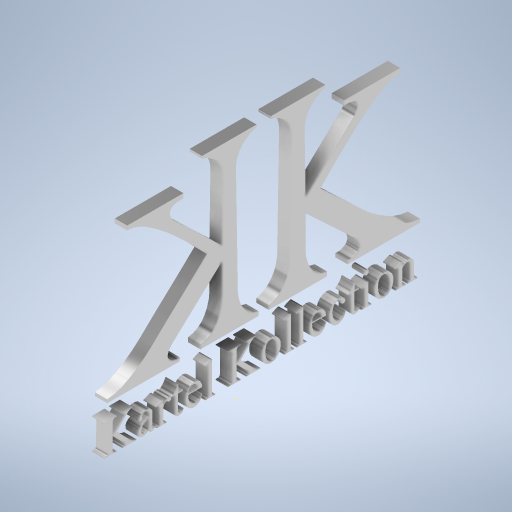
# Autodesk Inventor part: Kartel
Saved by Autodesk Inventor 2024 (Build 280153000, 153)
## iProperties
Created: 2024-08-29
Part Number: Kartel
Material: Genérico
Document SubType Name: Modeling
Designer: aless
Density: 1 g/cm^3
Appearance: Valor por defecto
Author: aless
Autodesk Inventor part; units mm, degrees
ref_plane "YZ Plane" through (0, 0, 0) normal (1, 0, 0) x (0, 1, 0)
ref_plane "XZ Plane" through (0, 0, 0) normal (0, 1, 0) x (-1, 0, 0)
ref_plane "XY Plane" through (0, 0, 0) normal (0, 0, 1) x (1, 0, 0)
sketch "Boceto1" plane through (0, 0, 0) normal (1, 0, 0) x (0, 1, 0)
  line L0 (223.396, 155.4576) -> (223.396, -178.2855) construction
  line L1 (223.396, -178.2855) -> (-110.3471, -178.2855) construction
  line L2 (-110.3471, -178.2855) -> (-110.3471, 155.4576) construction
  line L3 (-110.3471, 155.4576) -> (223.396, 155.4576) construction
  line L4 (59.7919, 115.7755) -> (59.7919, 56.339)
  line L5 (59.7919, 56.339) -> (62.7617, 56.339)
  arc A0 (64.6613, 64.2665) -> (62.7617, 56.339) centre (72.9401, 58.0914) ccw
  arc A1 (69.206, 66.1601) -> (64.6613, 64.2665) centre (68.5307, 61.3804) ccw
  arc A2 (72.0463, 65.151) -> (69.206, 66.1601) centre (68.1498, 58.6851) ccw
  arc A3 (76.4937, 61.3804) -> (72.0463, 65.151) centre (62.6533, 49.5641) ccw
  line L6 (76.4937, 61.3804) -> (113.4232, 21.7725)
  line L7 (113.4232, 21.7725) -> (88.008, 21.7725)
  arc A4 (71.6292, 26.2448) -> (88.008, 21.7725) centre (88.008, 54.0005) ccw
  arc A5 (63.3483, 39.331) -> (71.6292, 26.2448) centre (80.259, 40.8688) ccw
  line L8 (63.3483, 39.331) -> (59.7919, 39.331)
  line L9 (59.7919, 39.331) -> (59.7919, -8.3342)
  line L10 (59.7919, -8.3342) -> (63.1296, -8.3342)
  arc A6 (68.7765, 1.9584) -> (63.1296, -8.3342) centre (81.2261, -11.5671) ccw
  arc A7 (78.8624, 7.5023) -> (68.7765, 1.9584) centre (85.0773, -15.7512) ccw
  arc A8 (85.9805, 8.7127) -> (78.8624, 7.5023) centre (88.9297, -30.165) ccw
  line L11 (85.9805, 8.7127) -> (173.9872, 10.2175)
  arc A9 (184.4936, 7.5023) -> (173.9872, 10.2175) centre (174.3349, -10.1219) ccw
  arc A10 (194.6699, -6.6902) -> (184.4936, 7.5023) centre (173.2187, -11.3266) ccw
  line L12 (194.6699, -6.6902) -> (196.5458, -6.6902)
  line L13 (196.5458, -6.6902) -> (196.5458, 38.0381)
  line L14 (196.5458, 38.0381) -> (194.6699, 38.0381)
  arc A11 (186.9942, 25.7984) -> (194.6699, 38.0381) centre (168.397, 45.9875) ccw
  arc A12 (178.5832, 21.5693) -> (186.9942, 25.7984) centre (172.938, 43.2753) ccw
  arc A13 (175.6544, 21.0123) -> (178.5832, 21.5693) centre (172.938, 43.2753) ccw
  line L15 (175.6544, 21.0123) -> (124.7977, 21.7725)
  line L16 (124.7977, 21.7725) -> (161.7029, 60.4981)
  arc A14 (168.397, 64.5278) -> (161.7029, 60.4981) centre (170.5786, 53.329) ccw
  arc A15 (173.3252, 61.0636) -> (168.397, 64.5278) centre (168.6661, 59.673) ccw
  arc A16 (173.9954, 53.3315) -> (173.3252, 61.0636) centre (154.9336, 55.5745) ccw
  line L17 (173.9954, 53.3315) -> (177.7934, 53.3315)
  line L18 (177.7934, 53.3315) -> (177.7934, 99.4261)
  line L19 (177.7934, 99.4261) -> (174.3349, 99.4261)
  arc A17 (172.6788, 91.0496) -> (174.3349, 99.4261) centre (150.1011, 99.8653) ccw
  arc A18 (166.5655, 79.9474) -> (172.6788, 91.0496) centre (127.5163, 108.6838) ccw
  arc A19 (152.2652, 61.8267) -> (166.5655, 79.9474) centre (37.6495, 166.9808) ccw
  arc A20 (124.9813, 34.0587) -> (152.2652, 61.8267) centre (-154.1606, 335.6217) ccw
  arc A21 (95.3768, 65.5592) -> (124.9813, 34.0587) centre (1804.822, 1642.4536) ccw
  line L20 (95.3768, 65.5592) -> (82.3934, 79.0506)
  arc A22 (68.1498, 98.3694) -> (82.3934, 79.0506) centre (151.211, 144.6993) ccw
  arc A23 (62.5253, 115.7755) -> (68.1498, 98.3694) centre (101.6273, 118.7989) ccw
  line L21 (59.7919, 115.7755) -> (62.5253, 115.7755)
  line L22 (59.7919, -140.8555) -> (59.7919, -81.419)
  line L23 (59.7919, -81.419) -> (62.7617, -81.419)
  arc A24 (62.7617, -81.419) -> (64.6613, -89.3466) centre (72.9401, -83.1714) ccw
  arc A25 (64.6613, -89.3466) -> (69.206, -91.2401) centre (68.5307, -86.4604) ccw
  arc A26 (69.206, -91.2401) -> (72.0463, -90.231) centre (68.1498, -83.7652) ccw
  arc A27 (72.0463, -90.231) -> (76.4937, -86.4604) centre (62.6533, -74.6442) ccw
  line L24 (76.4937, -86.4604) -> (113.4232, -46.8526)
  line L25 (113.4232, -46.8526) -> (88.008, -46.8526)
  arc A28 (88.008, -46.8526) -> (71.6292, -51.3249) centre (88.008, -79.0805) ccw
  arc A29 (71.6292, -51.3249) -> (63.3483, -64.411) centre (80.259, -65.9489) ccw
  line L26 (63.3483, -64.411) -> (59.7919, -64.411)
  line L27 (59.7919, -64.411) -> (59.7919, -16.7458)
  line L28 (59.7919, -16.7458) -> (63.1296, -16.7458)
  arc A30 (63.1296, -16.7458) -> (68.7765, -27.0385) centre (81.2261, -13.513) ccw
  arc A31 (68.7765, -27.0385) -> (78.8624, -32.5823) centre (85.0773, -9.3289) ccw
  arc A32 (78.8624, -32.5823) -> (85.9805, -33.7928) centre (88.9297, 5.0849) ccw
  line L29 (85.9805, -33.7928) -> (173.9872, -35.2975)
  arc A33 (173.9872, -35.2975) -> (184.4936, -32.5823) centre (174.3349, -14.9582) ccw
  arc A34 (184.4936, -32.5823) -> (194.6699, -18.3898) centre (173.2187, -13.7535) ccw
  line L30 (194.6699, -18.3898) -> (196.5458, -18.3898)
  line L31 (196.5458, -18.3898) -> (196.5458, -63.1181)
  line L32 (196.5458, -63.1181) -> (194.6699, -63.1181)
  arc A35 (194.6699, -63.1181) -> (186.9942, -50.8784) centre (168.397, -71.0676) ccw
  arc A36 (186.9942, -50.8784) -> (178.5832, -46.6493) centre (172.938, -68.3554) ccw
  arc A37 (178.5832, -46.6493) -> (175.6544, -46.0923) centre (172.938, -68.3554) ccw
  line L33 (175.6544, -46.0923) -> (124.7977, -46.8526)
  line L34 (124.7977, -46.8526) -> (161.7029, -85.5781)
  arc A38 (161.7029, -85.5781) -> (168.397, -89.6078) centre (170.5786, -78.409) ccw
  arc A39 (168.397, -89.6078) -> (173.3252, -86.1436) centre (168.6661, -84.7531) ccw
  arc A40 (173.3252, -86.1436) -> (173.9954, -78.4115) centre (154.9336, -80.6545) ccw
  line L35 (173.9954, -78.4115) -> (177.7934, -78.4115)
  line L36 (177.7934, -78.4115) -> (177.7934, -124.5062)
  line L37 (177.7934, -124.5062) -> (174.3349, -124.5062)
  arc A41 (174.3349, -124.5062) -> (172.6788, -116.1296) centre (150.1011, -124.9454) ccw
  arc A42 (172.6788, -116.1296) -> (166.5655, -105.0274) centre (127.5163, -133.7638) ccw
  arc A43 (166.5655, -105.0274) -> (152.2652, -86.9067) centre (37.6495, -192.0609) ccw
  arc A44 (152.2652, -86.9067) -> (124.9813, -59.1387) centre (-154.1606, -360.7017) ccw
  arc A45 (124.9813, -59.1387) -> (95.3768, -90.6393) centre (1804.822, -1667.5336) ccw
  line L38 (95.3768, -90.6393) -> (82.3934, -104.1306)
  arc A46 (82.3934, -104.1306) -> (68.1498, -123.4494) centre (151.211, -169.7794) ccw
  arc A47 (68.1498, -123.4494) -> (62.5253, -140.8555) centre (101.6273, -143.879) ccw
  line L39 (59.7919, -140.8555) -> (62.5253, -140.8555)
  arc A48 (38.0866, 85.5965) -> (35.5198, 87.3022) centre (35.8691, 85.0436) ccw
  arc A49 (36.8943, 82.0362) -> (38.0866, 85.5965) centre (34.9982, 84.651) ccw
  arc A50 (34.9982, 81.6224) -> (36.8943, 82.0362) centre (35.1843, 85.3209) ccw
  line L40 (34.9982, 81.6224) -> (32.9082, 81.6224)
  arc A51 (32.9082, 81.6224) -> (29.9007, 88.3728) centre (12.5435, 76.5945) ccw
  arc A52 (29.9007, 88.3728) -> (24.2156, 90.5789) centre (25.542, 85.5688) ccw
  arc A53 (24.2156, 90.5789) -> (21.9144, 84.651) centre (25.5922, 86.6339) ccw
  arc A54 (21.9144, 84.651) -> (24.2156, 81.6224) centre (39.6273, 95.7211) ccw
  arc A55 (23.3542, 81.4464) -> (24.2156, 81.6224) centre (23.3384, 83.7198) ccw
  arc A56 (23.3542, 81.4464) -> (21.6972, 78.3656) centre (23.3681, 79.4529) ccw
  arc A57 (21.6972, 78.3656) -> (24.0265, 75.8904) centre (29.735, 83.5959) ccw
  line L41 (24.0265, 75.8904) -> (24.977, 75.8904)
  arc A58 (23.7493, 77.1285) -> (24.977, 75.8904) centre (26.642, 78.769) ccw
  arc A59 (24.5577, 78.769) -> (23.7493, 77.1285) centre (24.9399, 77.5613) ccw
  line L42 (24.5577, 78.769) -> (34.6579, 78.769)
  arc A60 (34.6579, 78.769) -> (36.5914, 78.9939) centre (35.1641, 82.8408) ccw
  arc A61 (36.5914, 78.9939) -> (38.1207, 80.244) centre (34.9292, 82.5878) ccw
  arc A62 (38.1207, 80.244) -> (39.1394, 82.8837) centre (33.769, 83.4399) ccw
  arc A63 (39.1394, 82.8837) -> (39.1713, 85.2713) centre (22.5869, 84.2987) ccw
  arc A64 (39.1713, 85.2713) -> (37.0863, 89.3907) centre (33.3893, 84.9322) ccw
  arc A65 (37.0863, 89.3907) -> (34.4999, 89.9538) centre (35.1334, 86.6421) ccw
  arc A66 (34.4999, 89.9538) -> (33.5882, 87.7349) centre (34.6764, 88.5846) ccw
  arc A67 (33.5882, 87.7349) -> (35.5198, 87.3022) centre (34.8398, 88.794) ccw
  line L43 (31.9452, 81.6224) -> (25.277, 81.6224)
  arc A68 (23.3681, 85.4937) -> (25.277, 81.6224) centre (28.802, 85.7668) ccw
  arc A69 (25.3794, 87.7349) -> (23.3681, 85.4937) centre (25.602, 85.5121) ccw
  arc A70 (29.6078, 86.2704) -> (25.3794, 87.7349) centre (26.3335, 83.6533) ccw
  arc A71 (31.9452, 81.6224) -> (29.6078, 86.2704) centre (15.4947, 76.2615) ccw
  line L44 (21.6124, 75.123) -> (21.6124, 66.9623)
  line L45 (21.6124, 66.9623) -> (22.1976, 66.9623)
  arc A72 (23.8036, 69.605) -> (22.1976, 66.9623) centre (24.42, 67.421) ccw
  arc A73 (25.0547, 69.7635) -> (23.8036, 69.605) centre (24.8387, 66.4503) ccw
  line L46 (25.0547, 69.7635) -> (33.686, 69.7635)
  arc A74 (36.3591, 68.1202) -> (33.686, 69.7635) centre (33.1882, 65.9579) ccw
  arc A75 (36.4721, 66.3785) -> (36.3591, 68.1202) centre (35.0858, 67.1631) ccw
  arc A76 (36.4721, 66.3785) -> (36.1827, 63.6509) centre (37.3383, 64.9074) ccw
  arc A77 (36.1827, 63.6509) -> (38.546, 63.7009) centre (37.3383, 64.9074) ccw
  arc A78 (38.546, 63.7009) -> (38.8749, 66.6601) centre (36.4741, 65.429) ccw
  arc A79 (38.8749, 66.6601) -> (35.5198, 69.4394) centre (32.3716, 62.2244) ccw
  arc A80 (35.5198, 69.7635) -> (35.5198, 69.4394) centre (35.6479, 69.6014) ccw
  line L47 (35.5198, 69.7635) -> (39.1779, 69.7635)
  line L48 (39.1779, 69.7635) -> (39.1779, 71.1938)
  line L49 (39.1779, 71.1938) -> (37.1902, 75.9142)
  line L50 (37.1902, 75.9142) -> (36.655, 75.9142)
  arc A81 (36.2727, 73.4734) -> (36.655, 75.9142) centre (34.9055, 74.9378) ccw
  arc A82 (35.4631, 73.138) -> (36.2727, 73.4734) centre (35.236, 74.8315) ccw
  line L51 (35.4631, 73.138) -> (23.8203, 72.7044)
  arc A83 (22.4058, 73.9437) -> (23.8203, 72.7044) centre (23.8947, 74.2162) ccw
  line L52 (22.4058, 73.9437) -> (22.3522, 75.123)
  line L53 (22.3522, 75.123) -> (21.6124, 75.123)
  line L54 (38.1207, 62.9191) -> (37.6239, 62.9191)
  arc A84 (38.1207, 62.9191) -> (44.215, 58.0655) centre (46.9664, 67.7732) ccw
  line L55 (44.215, 58.0655) -> (44.215, 57.4949)
  line L56 (44.215, 57.4949) -> (38.546, 57.4949)
  line L57 (38.546, 57.4949) -> (38.546, 53.7418)
  line L58 (38.546, 53.7418) -> (37.6239, 53.7418)
  line L59 (37.6239, 53.7418) -> (37.6239, 57.6656)
  line L60 (37.6239, 57.6656) -> (25.9541, 57.6656)
  arc A85 (25.9541, 57.6656) -> (24.0759, 57.0554) centre (25.6588, 55.3787) ccw
  arc A86 (24.0759, 57.0554) -> (24.0759, 54.3896) centre (25.4621, 55.7225) ccw
  arc A87 (24.0759, 54.3896) -> (24.977, 53.7418) centre (26.9231, 57.3995) ccw
  line L61 (24.977, 53.7418) -> (24.977, 53.123)
  arc A88 (21.9823, 58.8624) -> (24.977, 53.123) centre (25.6258, 57.1125) ccw
  arc A89 (25.4621, 60.3359) -> (21.9823, 58.8624) centre (24.8526, 56.9298) ccw
  line L62 (25.4621, 60.3359) -> (37.6239, 60.3359)
  line L63 (37.6239, 60.3359) -> (37.6239, 62.9191)
  line L64 (32.3716, 49.3309) -> (32.3716, 37.9509)
  arc A90 (32.3716, 37.9509) -> (38.546, 41.305) centre (32.9408, 44.2631) ccw
  arc A91 (38.546, 41.305) -> (38.8321, 46.6) centre (32.9408, 44.2631) ccw
  arc A92 (38.8321, 46.6) -> (33.9054, 51.0491) centre (31.015, 42.8962) ccw
  arc A93 (33.9054, 51.0491) -> (25.4621, 50.8397) centre (29.9574, 39.913) ccw
  arc A94 (25.4621, 50.8397) -> (21.373, 45.7244) centre (28.4076, 44.293) ccw
  arc A95 (21.373, 45.7244) -> (24.6427, 39.0414) centre (27.4289, 44.546) ccw
  arc A96 (24.6427, 39.0414) -> (27.8582, 37.816) centre (29.5234, 47.0167) ccw
  line L65 (27.8582, 37.816) -> (28.1489, 38.3827)
  arc A97 (24.2156, 44.1766) -> (28.1489, 38.3827) centre (29.1956, 43.3253) ccw
  arc A98 (32.3716, 49.3309) -> (24.2156, 44.1766) centre (31.2116, 42.1364) ccw
  line L66 (33.3994, 49.3309) -> (33.3994, 41.5084)
  arc A99 (33.3994, 41.5084) -> (37.9867, 45.2157) centre (33.8115, 45.6901) ccw
  arc A100 (37.9867, 45.2157) -> (33.3994, 49.3309) centre (33.9488, 45.3289) ccw
  line L67 (21.6124, 35.3726) -> (21.6124, 27.2167)
  line L68 (21.6124, 27.2167) -> (22.1976, 27.2167)
  arc A101 (24.0759, 29.9109) -> (22.1976, 27.2167) centre (24.3353, 27.7281) ccw
  line L69 (24.0759, 29.9109) -> (48.1783, 29.9109)
  line L70 (48.1783, 29.9109) -> (48.1783, 30.6705)
  line L71 (48.1783, 30.6705) -> (46.1559, 35.5025)
  line L72 (46.1559, 35.5025) -> (45.435, 35.2832)
  arc A102 (44.9538, 32.9704) -> (45.435, 35.2832) centre (44.1811, 34.3376) ccw
  line L73 (44.9538, 32.9704) -> (23.8947, 32.9704)
  arc A103 (22.3522, 35.2151) -> (23.8947, 32.9704) centre (24.0502, 34.7296) ccw
  line L74 (21.6124, 35.3726) -> (22.3522, 35.3726)
  line L75 (22.3522, 35.3726) -> (22.3522, 35.2151)
  line L76 (21.6124, 16.6489) -> (21.6124, 6.2709)
  line L77 (21.6124, 6.2709) -> (22.1976, 6.2709)
  arc A104 (23.1319, 9.3747) -> (22.1976, 6.2709) centre (25.372, 7.0079) ccw
  arc A105 (24.083, 9.6851) -> (23.1319, 9.3747) centre (23.9349, 8.5262) ccw
  line L78 (24.083, 9.6851) -> (34.4242, 9.6851)
  line L79 (34.4242, 9.6851) -> (24.6427, 0.2674)
  arc A106 (22.5322, 0.2674) -> (24.6427, 0.2674) centre (23.5875, 1.1984) ccw
  arc A107 (22.3385, 1.8467) -> (22.5322, 0.2674) centre (24.1733, 1.2702) ccw
  line L80 (22.3385, 1.8467) -> (21.6972, 1.8467)
  line L81 (21.6972, 1.8467) -> (21.6972, -9.7309)
  line L82 (21.6972, -9.7309) -> (22.1976, -9.7309)
  arc A108 (25.4621, -3.6316) -> (22.1976, -9.7309) centre (30.676, -10.3456) ccw
  arc A109 (35.6479, 6.2709) -> (25.4621, -3.6316) centre (530.6587, -513.089) ccw
  line L83 (35.6479, 6.2709) -> (43.5185, -1.3435)
  arc A110 (45.6956, -3.8414) -> (43.5185, -1.3435) centre (36.8132, -9.385) ccw
  arc A111 (46.3952, -6.3342) -> (45.6956, -3.8414) centre (40.9755, -6.5108) ccw
  line L84 (46.3952, -6.3342) -> (46.9664, -6.3342)
  line L85 (46.9664, -6.3342) -> (46.9664, 2.4637)
  line L86 (46.9664, 2.4637) -> (46.3563, 2.4637)
  arc A112 (46.038, 0.6299) -> (46.3563, 2.4637) centre (44.4623, 1.8479) ccw
  arc A113 (44.1033, 0.4662) -> (46.038, 0.6299) centre (44.9765, 1.66) ccw
  line L87 (44.1033, 0.4662) -> (34.7864, 9.6369)
  line L88 (34.7864, 9.6369) -> (44.4623, 9.6369)
  arc A114 (46.2145, 8.4652) -> (44.4623, 9.6369) centre (44.3645, 7.5946) ccw
  arc A115 (46.3563, 6.3777) -> (46.2145, 8.4652) centre (42.3519, 7.1543) ccw
  line L89 (46.3563, 6.3777) -> (46.9231, 6.3777)
  line L90 (46.9231, 6.3777) -> (46.9231, 16.6489)
  line L91 (46.9231, 16.6489) -> (46.3563, 16.6489)
  arc A116 (46.038, 14.2838) -> (46.3563, 16.6489) centre (41.1694, 16.143) ccw
  arc A117 (44.9101, 13.1919) -> (46.038, 14.2838) centre (44.3089, 14.9413) ccw
  arc A118 (43.9559, 13.0395) -> (44.9101, 13.1919) centre (43.2415, 20.5755) ccw
  line L92 (43.9559, 13.0395) -> (23.9783, 13.1915)
  arc A119 (22.3385, 14.7793) -> (23.9783, 13.1915) centre (23.9909, 14.8452) ccw
  line L93 (22.3385, 14.7793) -> (22.3385, 16.6489)
  line L94 (22.3385, 16.6489) -> (21.6124, 16.6489)
  arc A120 (38.9559, -20.635) -> (38.546, -15.7512) centre (32.1503, -18.7471) ccw
  arc A121 (29.735, -26.5419) -> (38.9559, -20.635) centre (30.7842, -18.0292) ccw
  arc A122 (24.0186, -24.2681) -> (29.735, -26.5419) centre (30.5703, -16.1196) ccw
  arc A123 (21.2736, -18.7471) -> (24.0186, -24.2681) centre (28.6304, -18.5322) ccw
  arc A124 (24.7689, -12.2667) -> (21.2736, -18.7471) centre (28.6304, -18.5322) ccw
  arc A125 (31.3501, -10.8287) -> (24.7689, -12.2667) centre (30.1103, -20.9334) ccw
  arc A126 (38.546, -15.7512) -> (31.3501, -10.8287) centre (30.893, -19.2177) ccw
  arc A127 (36.6462, -21.2165) -> (36.4528, -15.186) centre (34.1039, -18.2797) ccw
  arc A128 (31.6291, -23.1781) -> (36.6462, -21.2165) centre (30.802, -13.6656) ccw
  arc A129 (26.7058, -23.1781) -> (31.6291, -23.1781) centre (29.1675, -1.1021) ccw
  arc A130 (24.1733, -22.2544) -> (26.7058, -23.1781) centre (27.2468, -17.7612) ccw
  arc A131 (23.3681, -16.5877) -> (24.1733, -22.2544) centre (26.3634, -19.0526) ccw
  arc A132 (29.9007, -13.9628) -> (23.3681, -16.5877) centre (29.8882, -23.3729) ccw
  arc A133 (34.2789, -14.2432) -> (29.9007, -13.9628) centre (31.1362, -28.9932) ccw
  arc A134 (36.4528, -15.186) -> (34.2789, -14.2432) centre (33.7557, -18.4271) ccw
  line L95 (24.0759, -34.8591) -> (48.1783, -34.8591)
  line L96 (44.9538, -31.7996) -> (23.8947, -31.7996)
  arc A135 (44.9538, -31.7996) -> (45.435, -29.4868) centre (44.1811, -30.4324) ccw
  line L97 (46.1559, -29.2675) -> (45.435, -29.4868)
  line L98 (48.1783, -34.0995) -> (46.1559, -29.2675)
  line L99 (48.1783, -34.8591) -> (48.1783, -34.0995)
  arc A136 (22.3522, -29.5549) -> (23.8947, -31.7996) centre (24.0502, -30.0404) ccw
  line L100 (21.6124, -29.3974) -> (22.3522, -29.3974)
  line L101 (22.3522, -29.3974) -> (22.3522, -29.5549)
  line L102 (21.6124, -29.3974) -> (21.6124, -37.5533)
  line L103 (21.6124, -37.5533) -> (22.1976, -37.5533)
  arc A137 (24.0759, -34.8591) -> (22.1976, -37.5533) centre (24.3353, -37.0419) ccw
  line L104 (44.9538, -41.9596) -> (23.8947, -41.9596)
  arc A138 (44.9538, -41.9596) -> (45.435, -39.6468) centre (44.1811, -40.5924) ccw
  line L105 (46.1559, -39.4275) -> (45.435, -39.6468)
  line L106 (48.1783, -44.2595) -> (46.1559, -39.4275)
  line L107 (48.1783, -45.0191) -> (48.1783, -44.2595)
  line L108 (24.0759, -45.0191) -> (48.1783, -45.0191)
  arc A139 (24.0759, -45.0191) -> (22.1976, -47.7133) centre (24.3353, -47.2019) ccw
  arc A140 (22.3522, -39.7149) -> (23.8947, -41.9596) centre (24.0502, -40.2004) ccw
  line L109 (22.3522, -39.5574) -> (22.3522, -39.7149)
  line L110 (21.6124, -39.5574) -> (22.3522, -39.5574)
  line L111 (21.6124, -39.5574) -> (21.6124, -47.7133)
  line L112 (21.6124, -47.7133) -> (22.1976, -47.7133)
  line L113 (32.3716, -52.2691) -> (32.3716, -63.6491)
  line L114 (33.3994, -52.2691) -> (33.3994, -60.0916)
  arc A141 (33.3994, -60.0916) -> (37.9867, -56.3843) centre (33.8115, -55.9099) ccw
  arc A142 (37.9867, -56.3843) -> (33.3994, -52.2691) centre (33.9488, -56.2711) ccw
  arc A143 (32.3716, -63.6491) -> (38.546, -60.295) centre (32.9408, -57.3369) ccw
  arc A144 (38.546, -60.295) -> (38.8321, -55) centre (32.9408, -57.3369) ccw
  arc A145 (38.8321, -55) -> (33.9054, -50.5509) centre (31.015, -58.7038) ccw
  arc A146 (33.9054, -50.5509) -> (25.4621, -50.7603) centre (29.9574, -61.687) ccw
  arc A147 (25.4621, -50.7603) -> (21.373, -55.8756) centre (28.4076, -57.307) ccw
  arc A148 (21.373, -55.8756) -> (24.6427, -62.5586) centre (27.4289, -57.054) ccw
  arc A149 (24.6427, -62.5586) -> (27.8582, -63.784) centre (29.5234, -54.5833) ccw
  line L115 (27.8582, -63.784) -> (28.1489, -63.2173)
  arc A150 (24.2156, -57.4234) -> (28.1489, -63.2173) centre (29.1956, -58.2747) ccw
  arc A151 (32.3716, -52.2691) -> (24.2156, -57.4234) centre (31.2116, -59.4636) ccw
  arc A152 (35.9662, -75.927) -> (33.9054, -78.5277) centre (35.7126, -77.8429) ccw
  arc A153 (38.6103, -71.1233) -> (34.4237, -66.9057) centre (31.1389, -74.353) ccw
  arc A154 (22.6462, -69.4024) -> (22.1976, -76.1864) centre (26.8574, -73.0877) ccw
  arc A155 (22.1976, -76.1864) -> (28.0565, -80.0142) centre (29.2604, -71.7737) ccw
  line L116 (28.0565, -80.0142) -> (28.3058, -79.4786)
  arc A156 (34.8518, -69.4605) -> (31.1389, -68.9129) centre (31.4763, -79.4858) ccw
  arc A157 (38.0849, -72.7596) -> (34.8518, -69.4605) centre (33.6168, -73.9046) ccw
  arc A158 (37.6239, -75.2191) -> (38.0849, -72.7596) centre (34.9678, -73.4483) ccw
  arc A159 (35.9662, -75.927) -> (37.6239, -75.2191) centre (36.1145, -73.9794) ccw
  line L117 (37.6239, -84.1901) -> (37.6239, -81.6069)
  line L118 (38.1207, -81.6069) -> (37.6239, -81.6069)
  arc A160 (38.1207, -81.6069) -> (44.215, -86.4605) centre (46.9664, -76.7528) ccw
  line L119 (44.215, -86.4605) -> (44.215, -87.0311)
  line L120 (44.215, -87.0311) -> (38.546, -87.0311)
  line L121 (38.546, -87.0311) -> (38.546, -90.7842)
  line L122 (38.546, -90.7842) -> (37.6239, -90.7842)
  line L123 (37.6239, -90.7842) -> (37.6239, -86.8604)
  line L124 (37.6239, -86.8604) -> (25.9541, -86.8604)
  arc A161 (25.9541, -86.8604) -> (24.0759, -87.4706) centre (25.6588, -89.1473) ccw
  arc A162 (24.0759, -87.4706) -> (24.0759, -90.1364) centre (25.4621, -88.8035) ccw
  arc A163 (24.0759, -90.1364) -> (24.977, -90.7842) centre (26.9231, -87.1265) ccw
  line L125 (24.977, -90.7842) -> (24.977, -91.403)
  arc A164 (21.9823, -85.6636) -> (24.977, -91.403) centre (25.6258, -87.4135) ccw
  arc A165 (25.4621, -84.1901) -> (21.9823, -85.6636) centre (24.8526, -87.5962) ccw
  line L126 (25.4621, -84.1901) -> (37.6239, -84.1901)
  line L127 (21.6124, -92.7349) -> (21.6124, -100.8569)
  line L128 (21.6124, -100.8569) -> (22.3522, -100.8569)
  arc A166 (23.7493, -98.4636) -> (22.3522, -100.8569) centre (24.1957, -100.3286) ccw
  line L129 (23.7493, -98.4636) -> (39.2417, -98.4636)
  line L130 (39.2417, -98.4636) -> (39.2417, -97.3849)
  line L131 (39.2417, -97.3849) -> (37.1902, -92.5811)
  line L132 (37.1902, -92.5811) -> (36.4528, -92.8209)
  arc A167 (35.7582, -95.2926) -> (36.4528, -92.8209) centre (35.3013, -93.8308) ccw
  line L133 (35.7582, -95.2926) -> (23.7493, -95.2926)
  arc A168 (22.4058, -93.5527) -> (23.7493, -95.2926) centre (23.9167, -93.7747) ccw
  line L134 (22.4058, -93.5527) -> (22.4058, -92.7349)
  line L135 (22.4058, -92.7349) -> (21.6124, -92.7349)
  circle A169 centre (46.3343, -96.7959) radius 1.9807
  arc A170 (29.9007, -106.4188) -> (23.3681, -109.0437) centre (29.8882, -115.8289) ccw
  arc A171 (23.3681, -109.0437) -> (24.1733, -114.7104) centre (26.3634, -111.5086) ccw
  arc A172 (24.1733, -114.7104) -> (26.7058, -115.6341) centre (27.2468, -110.2172) ccw
  arc A173 (26.7058, -115.6341) -> (31.6291, -115.6341) centre (29.1675, -93.5581) ccw
  arc A174 (31.6291, -115.6341) -> (36.6462, -113.6725) centre (30.802, -106.1216) ccw
  arc A175 (36.6462, -113.6725) -> (36.4528, -107.642) centre (34.1039, -110.7357) ccw
  arc A176 (36.4528, -107.642) -> (34.2789, -106.6992) centre (33.7557, -110.8831) ccw
  arc A177 (34.2789, -106.6992) -> (29.9007, -106.4188) centre (31.1362, -121.4492) ccw
  arc A178 (21.2736, -111.2031) -> (24.0186, -116.7241) centre (28.6304, -110.9882) ccw
  arc A179 (24.0186, -116.7241) -> (29.735, -118.9979) centre (30.5703, -108.5756) ccw
  arc A180 (29.735, -118.9979) -> (38.9559, -113.091) centre (30.7842, -110.4852) ccw
  arc A181 (38.9559, -113.091) -> (38.546, -108.2072) centre (32.1503, -111.2031) ccw
  arc A182 (38.546, -108.2072) -> (31.3501, -103.2847) centre (30.893, -111.6737) ccw
  arc A183 (31.3501, -103.2847) -> (24.7689, -104.7227) centre (30.1103, -113.3894) ccw
  arc A184 (24.7689, -104.7227) -> (21.2736, -111.2031) centre (28.6304, -110.9882) ccw
  line L136 (21.4888, -120.5781) -> (21.4888, -128.8858)
  line L137 (21.4888, -128.8858) -> (22.3522, -128.8858)
  arc A185 (23.7493, -126.1735) -> (22.3522, -128.8858) centre (24.0784, -128.059) ccw
  line L138 (23.7493, -126.1735) -> (34.4238, -126.1735)
  arc A186 (36.9461, -130.1287) -> (34.4238, -126.1735) centre (31.5883, -130.7636) ccw
  arc A187 (35.2302, -132.6705) -> (36.9461, -130.1287) centre (34.6148, -130.405) ccw
  line L139 (35.2302, -132.6705) -> (23.5875, -132.6705)
  arc A188 (22.3769, -131.1179) -> (23.5875, -132.6705) centre (23.798, -131.2581) ccw
  line L140 (22.3769, -131.1179) -> (22.3769, -130.405)
  line L141 (22.3769, -130.405) -> (21.4888, -130.405)
  line L142 (21.4888, -130.405) -> (21.5438, -138.4848)
  line L143 (21.5438, -138.4848) -> (22.2644, -138.4799)
  arc A189 (23.4402, -136.1448) -> (22.2644, -138.4799) centre (24.2945, -138.0386) ccw
  arc A190 (24.7689, -135.9599) -> (23.4402, -136.1448) centre (24.4774, -138.7316) ccw
  line L144 (24.7689, -135.9599) -> (34.4238, -135.9599)
  arc A191 (36.9461, -127.2554) -> (35.7582, -126.306) centre (21.6046, -145.2328) ccw
  line L145 (35.7582, -126.306) -> (39.2276, -126.306)
  line L146 (39.2276, -126.306) -> (39.2276, -125.2648)
  line L147 (39.2276, -125.2648) -> (37.1761, -120.4367)
  arc A192 (35.8757, -123.0898) -> (36.3457, -120.7895) centre (35.3175, -121.7776) ccw
  line L148 (35.8757, -123.0898) -> (23.8725, -123.0898)
  arc A193 (22.2642, -121.3452) -> (23.8725, -123.0898) centre (24.0002, -121.3584) ccw
  line L149 (22.2642, -121.3226) -> (22.2642, -120.5781)
  line L150 (21.6124, 118.2489) -> (21.6124, 107.8709)
  line L151 (22.3385, 118.2489) -> (21.6124, 118.2489)
  line L152 (22.3385, 116.3793) -> (22.3385, 118.2489)
  arc A194 (22.3385, 116.3793) -> (23.9783, 114.7915) centre (23.9909, 116.4452) ccw
  line L153 (43.9559, 114.6395) -> (23.9783, 114.7915)
  arc A195 (43.9559, 114.6395) -> (44.9101, 114.7919) centre (43.2415, 122.1755) ccw
  arc A196 (44.9101, 114.7919) -> (46.038, 115.8838) centre (44.3089, 116.5413) ccw
  arc A197 (46.038, 115.8838) -> (46.3563, 118.2489) centre (41.1694, 117.743) ccw
  line L154 (46.9231, 118.2489) -> (46.3563, 118.2489)
  line L155 (46.9231, 107.9777) -> (46.9231, 118.2489)
  line L156 (46.3563, 107.9777) -> (46.9231, 107.9777)
  arc A198 (46.3563, 107.9777) -> (46.2145, 110.0652) centre (42.3519, 108.7543) ccw
  arc A199 (46.2145, 110.0652) -> (44.4623, 111.2369) centre (44.3645, 109.1946) ccw
  line L157 (34.7864, 111.2369) -> (44.4623, 111.2369)
  line L158 (44.1033, 102.0662) -> (34.7864, 111.2369)
  arc A200 (44.1033, 102.0662) -> (46.038, 102.2299) centre (44.9765, 103.26) ccw
  arc A201 (46.038, 102.2299) -> (46.3563, 104.0637) centre (44.4623, 103.4479) ccw
  line L159 (46.9664, 104.0637) -> (46.3563, 104.0637)
  line L160 (46.9664, 95.2658) -> (46.9664, 104.0637)
  line L161 (46.3952, 95.2658) -> (46.9664, 95.2658)
  arc A202 (46.3952, 95.2658) -> (45.6956, 97.7586) centre (40.9755, 95.0892) ccw
  arc A203 (45.6956, 97.7586) -> (43.5185, 100.2565) centre (36.8132, 92.215) ccw
  line L162 (35.6479, 107.8709) -> (43.5185, 100.2565)
  arc A204 (35.6479, 107.8709) -> (25.4621, 97.9684) centre (530.6587, -411.489) ccw
  arc A205 (25.4621, 97.9684) -> (22.1976, 91.8691) centre (30.676, 91.2544) ccw
  line L163 (21.6972, 91.8691) -> (22.1976, 91.8691)
  line L164 (21.6972, 103.4467) -> (21.6972, 91.8691)
  line L165 (22.3385, 103.4467) -> (21.6972, 103.4467)
  arc A206 (22.3385, 103.4467) -> (22.5322, 101.8674) centre (24.1733, 102.8702) ccw
  arc A207 (22.5322, 101.8674) -> (24.6427, 101.8674) centre (23.5875, 102.7984) ccw
  line L166 (34.4242, 111.2851) -> (24.6427, 101.8674)
  line L167 (24.083, 111.2851) -> (34.4242, 111.2851)
  arc A208 (23.1319, 110.9747) -> (22.1976, 107.8709) centre (25.372, 108.6079) ccw
  arc A209 (24.083, 111.2851) -> (23.1319, 110.9747) centre (23.9349, 110.1262) ccw
  line L168 (21.6124, 107.8709) -> (22.1976, 107.8709)
  arc A210 (34.4237, -66.9057) -> (22.6462, -69.4024) centre (30.2012, -76.014) ccw
  arc A211 (31.1389, -68.9129) -> (24.4774, -72.1545) centre (31.0947, -77.2875) ccw
  arc A212 (24.4774, -72.1545) -> (24.3353, -76.2961) centre (28.5963, -74.369) ccw
  arc A213 (24.3353, -76.2961) -> (28.3058, -79.4786) centre (29.8815, -73.4449) ccw
  arc A214 (33.9054, -78.5277) -> (36.2727, -79.2985) centre (35.4375, -77.8428) ccw
  arc A215 (36.2727, -79.2985) -> (39.2699, -73.9794) centre (33.6028, -74.2901) ccw
  arc A216 (39.2699, -73.9794) -> (38.6103, -71.1233) centre (31.1389, -74.353) ccw
  arc A217 (34.4238, -135.9599) -> (36.9461, -127.2554) centre (33.7183, -131.0378) ccw
  arc A218 (37.1761, -120.4367) -> (36.3457, -120.7895) centre (37.7848, -123.0228) ccw
  line L169 (21.4888, -120.5781) -> (22.2642, -120.5781)
  line L170 (22.2642, -121.3226) -> (22.2642, -121.3452)
  point P0 (0, 0)
  dimension "d12" = 64.77
  dimension "d20" = 74.93
  dimension "d28" = 101.6
  dimension "d36" = 144.526
  dimension "d44" = 92.456
  dimension "d52" = 101.6
  constraints: 443 point on circle, 334 end point, 219 centre point, 33 horizontal, 28 perpendicular, 24 tangent, 22 vertical, 3 concentric, 1 parallel, 269 other
  measures "d12" distance of L69.start L95.start
  measures "d20" distance of L73.start L104.start
  measures "d28" distance of L64.start L113.start
  measures "d36" distance of L62.end L117.start
  measures "d44" distance of A132.centre A170.centre
  measures "d52" distance of L76.start L150.start
sketch "Boceto2" plane through (0, 0, 0) normal (1, 0, 0) x (0, 1, 0)
  point P0 (0, 0)
extrude "Extrusión1" add sketch "Boceto1" along normal blind 10.16 contours L21 A23 A22 L20 A21 A20 A19 A18 A17 L19 L18 L17 A16 A15 A14 L16 L15 A13 A12 A11 L14 L13 L12 A10 A9 L11 A8 A7 A6 L10 L9 L8 A5 A4 L7 L6 A3 A2 A1 A0 L5 L4 | L22 L23 A24 A25 A26 A27 L24 L25 A28 A29 L26 L27 L28 A30 A31 A32 L29 A33 A34 L30 L31 L32 A35 A36 A37 L33 L34 A38 A39 A40 L35 L36 L37 A41 A42 A43 A44 A45 L38 A46 A47 L39 | A48 A67 A66 A65 A64 A63 A62 A61 A60 L42 A59 A58 L41 A57 A56 A55 A54 A53 A52 A51 L40 A50 A49 | L53 L52 A83 L51 A82 A81 L50 L49 L48 L47 A80 A79 A78 A77 A76 A75 A74 L46 A73 A72 L45 L44 | A84 L55 L56 L57 L58 L59 L60 A85 A86 A87 L61 A88 A89 L62 L63 L54 | A98 A97 L65 A96 A95 A94 A93 A92 A91 A90 L64 | L74 L75 A103 L73 A102 L72 L71 L70 L69 A101 L68 L67 | L94 L93 A119 L92 A118 A117 A116 L91 L90 L89 A115 A114 L88 L87 A113 A112 L86 L85 L84 A111 A110 L83 A109 A108 L82 L81 L80 A107 A106 L79 L78 A105 A104 L77 L76 | A121 A122 A123 A124 A125 A126 A120 | A137 L103 L102 L100 L101 A136 L96 A135 L97 L98 L99 L95 | A138 L105 L106 L107 L108 A139 L112 L111 L110 L109 A140 L104 | A151 A150 L115 A149 A148 A147 A146 A145 A144 A143 L113 | L117 L118 A160 L119 L120 L121 L122 L123 L124 A161 A162 A163 L125 A164 A165 L126 | L135 L134 A168 L133 A167 L132 L131 L130 L129 A166 L128 L127 | A169 | A177 A176 A175 A174 A173 A172 A171 A170 | A184 A183 A182 A181 A180 A179 A178 | L151 L152 A194 L153 A195 A196 A197 L154 L155 L156 A198 A199 L157 L158 A200 A201 L159 L160 L161 A202 A203 L162 A204 A205 L163 L164 L165 A206 A207 L166 L167 A209 A208 L168 L150
extrude "Extrusión2" cut sketch "Boceto1" along normal blind 10.16 contours A177 A176 A175 A174 A173 A172 A171 A170
extrude "Extrusión3" add sketch "Boceto1" along normal blind 10.16 contours A159 A158 A157 A156 A211 A212 A213 L116 A155 A154 A210 A153 A216 A215 A214 A152
extrude "Extrusión4" add sketch "Boceto1" along normal blind 10.16 contours L169 L149 L170 A193 L148 A192 A218 L147 L146 L145 A191 A217 L144 A190 A189 L143 L142 L141 L140 A188 L139 A187 A186 L138 A185 L137 L136
